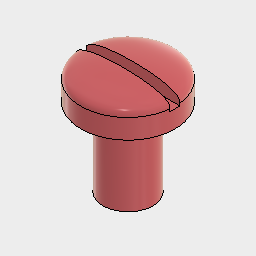
Test (Autodesk Fusion 360 archive; units mm, degrees)
design "BoltViaSaveObjectAs"
Autodesk Fusion 360 part; units mm, degrees
sketch "Sketch Profile" plane through (0, 0, 0) normal (0, -1, 0) x (1, 0, 0)
  line L0 (9.4718, -2.5516) -> (9.4718, -6.4965)
  line L1 (9.4718, -6.4965) -> (5, -6.4965)
  line L2 (5, -6.4965) -> (5, -22.1401)
  line L3 (5, -22.1401) -> (0, -22.1401)
  line L4 (0, -22.1401) -> (0, 0)
  spline S0 degree 5 poles (0, 0) (0.7576, 0) (2.2118, -0.0281) (4.2103, -0.1542) (6.4881, -0.471) (8.5163, -1.0493) (9.3202, -1.6158) (9.4718, -2.0782) (9.4718, -2.3938) (9.4718, -2.5516) knots 0 0 0 0 0 0 0.2 0.4 0.6 0.8 1 1 1 1 1 1
  line L5 (-2.0096, 0) -> (2.0096, 0)
  dimension "d14" = 5
  dimension "d22" = 0
  dimension "d23" = 0
  dimension "d24" = 0
  dimension "d25" = 0
  measures "d14" distance of L2.end L3.end
revolve "Revolve1" add sketch "Sketch Profile" angle 360 about axis through (0, 0, 1.75) along (0, 0, 1)
sketch "Sketch2" plane through (0, 0, 0) normal (0, 0, 1) x (1, 0, 0)
  line L0 (12.5, -1) -> (-12.5, -1)
  line L1 (-12.5, -1) -> (-12.5, 1)
  line L2 (-12.5, 1) -> (12.5, 1)
  line L3 (12.5, 1) -> (12.5, -1)
  line L4 (12.5, -1) -> (-12.5, 1) construction
  line L5 (-12.5, -1) -> (12.5, 1) construction
  dimension "d16" = 25
  dimension "d17" = 2
  measures "d16" distance of L0.start L0.end
  measures "d17" distance of L0.start L2.end
extrude "Extrude1" cut sketch "Sketch2" against normal blind 3
named bodies: "Bolt"

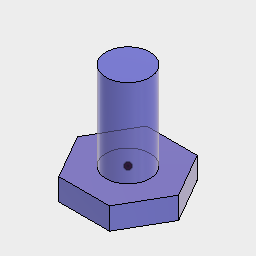
design "Bolt"
Autodesk Fusion 360 part; units mm, degrees
sketch "Sketch1" plane through (0, 0, 0) normal (0, 0, 1) x (1, 0, 0)
  circle A0 centre (0, 0) radius 5
  line L0 (5.7735, -10) -> (11.547, 0)
  line L1 (11.547, 0) -> (5.7735, 10)
  line L2 (5.7735, 10) -> (-5.7735, 10)
  line L3 (-5.7735, 10) -> (-11.547, 0)
  line L4 (-11.547, 0) -> (-5.7735, -10)
  line L5 (-5.7735, -10) -> (5.7735, -10)
  dimension "d1" = 10
  dimension "d2" = 10
  measures "d1" diameter of A0
  measures "d2" distance of A0.centre L5
extrude "Extrude1" add sketch "Sketch1" along normal blind 20 contours A0 makes body 1
extrude "Extrude2" add sketch "Sketch1" against normal blind 5 separate body contours A0 | L0 L1 L2 L3 L4 L5 makes body 2
